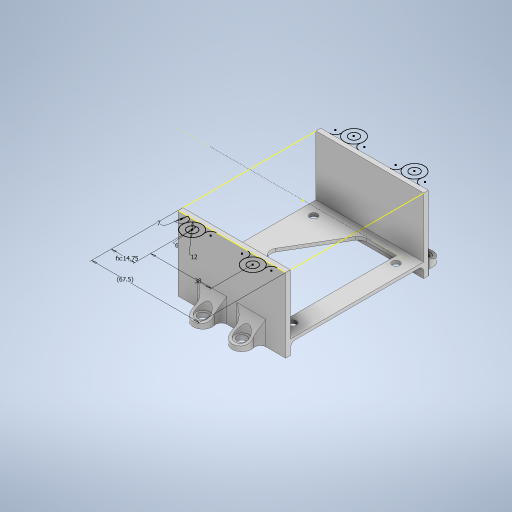
# Autodesk Inventor part: CO-1-02-fuseMount
Saved by Autodesk Inventor 2024 (Build 280153000, 153)
## iProperties
Created: 2023-03-23
Part Number: CO-1-02-fuseMount
Material: Generic
Document SubType Name: Modeling
Designer: beh5452
Density: 1 g/cm^3
Appearance: Default
Author: beh5452
Autodesk Inventor part; units mm, degrees
ref_plane "XZ Plane" through (0, 0, 0) normal (0, 1, 0) x (-1, 0, 0)
ref_plane "XY Plane" through (0, 0, 0) normal (0, 0, 1) x (1, 0, 0)
sketch "Sketch1" plane through (0, 0, 0) normal (0, 1, 0) x (-1, 0, 0)
  line L0 (33.75, 44.75) -> (-33.75, 44.75)
  line L1 (-33.75, 44.75) -> (-33.75, -44.75)
  line L2 (-33.75, -44.75) -> (33.75, -44.75)
  line L3 (33.75, -44.75) -> (33.75, 44.75)
  line L4 (21.75, -36.75) -> (-21.75, -36.75)
  line L5 (21.75, 36.75) -> (-21.75, 36.75)
  line L6 (21.75, 36.75) -> (21.75, -36.75)
  line L7 (-21.75, 36.75) -> (-21.75, -36.75)
  line L8 (33.75, -41.75) -> (-33.75, -41.75)
  line L9 (33.75, 41.75) -> (-33.75, 41.75)
  line L10 (-6.7955, 36.75) -> (21.75, 0)
  line L11 (21.75, 0) -> (0, -36.75)
  point P0 (0, 0)
  point P1 (-33.75, 0)
  dimension "d0" = 83.5
  dimension "d1" = 3
  dimension "d2" = 3
  dimension "d4" = 5
  dimension "d5" = 5
  dimension "d6" = 12
  dimension "d7" = 12
  dimension "d8" = 67.5
  dimension "d9" = 33.75
  dimension "d10" = 41.75
  constraints: 24 end point, 7 perpendicular, 5 point on line, 3 horizontal, 3 midpoint
  measures "d0" distance between parallel lines of L8 L9
  measures "d1" distance between parallel lines of L0 L9
  measures "d2" distance between parallel lines of L8 L2
  measures "d4" distance between parallel lines of L9 L5
  measures "d5" distance between parallel lines of L8 L4
  measures "d6" distance between parallel lines of L3 L6
  measures "d7" distance between parallel lines of L7 L1
  measures "d8" distance from line of point (-33.75, 0) L3
  measures "d9" distance from line of point (0, 0) L1
  measures "d10" distance from line of point (0, 0) L8
extrude "Extrusion1" add sketch "Sketch1" along normal blind 2 contours L3 L8 L1 L9 | L4 L11 L6 | L10 L5 L6
extrude "Extrusion2" add sketch "Sketch1" along normal blind 39.5 and the other way blind 7 contours L3 L9 L1 L0 | L3 L2 L1 L8
sketch "Sketch4" plane through (0, 2, 0) normal (0, 1, 0) x (1, 0, 0)
  circle A0 centre (-25.8, -32.4) radius 2.35
  circle A1 centre (-25.8, 32.4) radius 2.35
  circle A2 centre (25.8, -32.4) radius 2.35
  circle A3 centre (25.8, 32.4) radius 2.35
  line L0 (-33.75, 41.75) -> (-33.75, -41.75) projected
  line L1 (-33.75, -41.75) -> (33.75, -41.75) projected
  line L2 (33.75, -41.75) -> (33.75, 41.75) projected
  line L3 (33.75, 41.75) -> (-33.75, 41.75) projected
  point P0 (0, 0)
  dimension "d35" = 4.7
  dimension "d36" = 7.95
  dimension "d38" = 7.95
  dimension "d73" = 64.8
  dimension "d74" = 32.4
  constraints: 4 centre point, 3 equal radius, 2 horizontal alignment, 2 vertical alignment
  measures "d35" diameter of A0
  measures "d36" distance from line of L0 A0.centre
  measures "d38" distance from line of L2 A3.centre
  measures "d73" distance of A0.centre A1.centre
  measures "d74" vertical distance of point (0, 0) A0.centre
extrude "Extrusion6" cut sketch "Sketch4" against normal blind 3 contours A0 | A1 | A2 | A3
sketch "Sketch6" plane through (0, -7, 0) normal (0, -1, 0) x (1, 0, 0)
  circle A0 centre (-12.25, 50.75) radius 3
  circle A1 centre (12.25, 50.75) radius 3
  circle A2 centre (-24.5, -50.75) radius 3
  circle A3 centre (24.5, -50.75) radius 3
  circle A4 centre (-12.25, 50.75) radius 6
  circle A5 centre (-24.5, -50.75) radius 6
  circle A6 centre (24.5, -50.75) radius 6
  circle A7 centre (12.25, 50.75) radius 6
  arc A8 (-21.4152, 44.75) -> (-18.0385, 49.1711) centre (-21.4152, 48.25) ccw
  arc A9 (-6.4615, 49.1711) -> (-3.0848, 44.75) centre (-3.0848, 48.25) ccw
  arc A10 (3.0848, 44.75) -> (6.4615, 49.1711) centre (3.0848, 48.25) ccw
  arc A11 (18.0385, 49.1711) -> (21.4152, 44.75) centre (21.4152, 48.25) ccw
  arc A12 (-30.2885, -49.1711) -> (-33.6652, -44.75) centre (-33.6652, -48.25) ccw
  arc A13 (-15.3348, -44.75) -> (-18.7115, -49.1711) centre (-15.3348, -48.25) ccw
  arc A14 (18.7115, -49.1711) -> (15.3348, -44.75) centre (15.3348, -48.25) ccw
  arc A15 (33.6652, -44.75) -> (30.2885, -49.1711) centre (33.6652, -48.25) ccw
  line L0 (0, -79.45) -> (0, 79.45) projected
  circle A16 centre (0, -50.75) radius 3
  circle A17 centre (0, -50.75) radius 6
  arc A18 (9.1652, -44.75) -> (5.7885, -49.1711) centre (9.1652, -48.25) ccw
  arc A19 (-5.7885, -49.1711) -> (-9.1652, -44.75) centre (-9.1652, -48.25) ccw
  line L1 (-33.75, -44.75) -> (33.75, -44.75) projected
  line L2 (33.75, 44.75) -> (-33.75, 44.75) projected
  point P0 (0, 0)
  point P1 (-24.5, -44.75)
  point P2 (0, -44.75)
  point P3 (24.5, -44.75)
  point P4 (12.25, 44.75)
  point P5 (-12.25, 44.75)
  dimension "d46" = 6
  dimension "d47" = 6
  dimension "d48" = 6
  dimension "d49" = 6
  dimension "d51" = 12
  dimension "d54" = 3.5
  dimension "d55" = 24.5
  dimension "d56" = 49
  dimension "d57" = 12.25
  dimension "d58" = 24.5
  constraints: 30 point on circle, 25 tangent, 20 centre point, 14 equal radius, 5 coincident, 3 point on line
  measures "d46" diameter of A0
  measures "d47" diameter of A1
  measures "d48" diameter of A2
  measures "d49" diameter of A3
  measures "d51" diameter of A5
  measures "d54" radius of A12
  measures "d55" distance of A0.centre A1.centre
  measures "d56" distance of A3.centre A2.centre
  measures "d57" distance from line of L0 A1.centre
  measures "d58" distance from line of L0 A3.centre
extrude "Extrusion7" add sketch "Sketch6" against normal blind 15 contours A4 | A4 L2 A8 | A9 L2 A4 | A5 | A5 L1 A13 | A12 L1 A5 | A6 | A6 L1 A15 | A14 L1 A6 | A7 | A7 L2 A10 | A11 L2 A7 | A17 L0 A16 | L0 A16 A17 | A19 L1 A17 | L1 A18 A17
sketch "Sketch7" plane through (0, 8, 0) normal (0, 1, 0) x (1, 0, 0)
  circle A0 centre (-12.25, -50.75) radius 3 projected
  circle A1 centre (-12.25, -50.75) radius 4.25
  circle A2 centre (12.25, -50.75) radius 3 projected
  circle A3 centre (24.5, 50.75) radius 3 projected
  circle A4 centre (-24.5, 50.75) radius 3 projected
  circle A5 centre (12.25, -50.75) radius 3 projected
  circle A6 centre (12.25, -50.75) radius 4.25
  circle A7 centre (24.5, 50.75) radius 4.25
  circle A8 centre (-24.5, 50.75) radius 4.25
  circle A9 centre (0, 50.75) radius 3 projected
  circle A10 centre (0, 50.75) radius 4.25
  point P0 (0, 0)
  dimension "d61" = 8.5
  dimension "d62" = 8.5
  dimension "d63" = 8.5
  dimension "d64" = 8.5
  dimension "d72" = 8.5
  constraints: 5 centre point, 5 coincident
  measures "d61" diameter of A1
  measures "d62" diameter of A6
  measures "d63" diameter of A7
  measures "d64" diameter of A8
  measures "d72" diameter of A10
extrude "Extrusion8" cut sketch "Sketch7" against normal blind 12 contours A1 | A3 | A4 | A6 | A7 | A8 | A9 | A10
ref_plane "Work Plane1" through (30, 0, 0) normal (1, 0, 0) x (0, 1, 0)
sketch "Sketch8" plane through (30, 0, 0) normal (1, 0, 0) x (0, 1, 0)
  line L0 (-7, 56.75) -> (8, 56.75) projected
  line L1 (8, 49.1711) -> (8, 44.75) projected
  arc A0 (-4, 56.75) -> (8, 44.75) centre (8, 56.75) ccw
  line L2 (-7, 56.75) -> (-7, 44.75) projected
  line L3 (39.5, 44.75) -> (-7, 44.75) projected
  line L4 (8, 49.1711) -> (8, 56.75) projected
  arc A1 (8, -44.75) -> (-4, -56.75) centre (8, -56.75) ccw
  line L5 (8, -44.75) -> (8, -49.1711) projected
  line L6 (-7, -56.75) -> (8, -56.75) projected
  line L7 (-7, -49.1711) -> (-7, -56.75) projected
  line L8 (8, -46.5) -> (8, -55) projected
  line L9 (8, -56.75) -> (8, -49.1711) projected
  point P0 (0, 0)
  point P1 (42.5, 44.75)
  point P2 (-4, -56.75)
  dimension "d68" = 3
  dimension "d80" = 3
  constraints: 4 point on circle, 2 centre point, 1 point on line, 1 tangent
  measures "d68" distance from line of A0.start L2
  measures "d80" distance from line of L7 A1.end
extrude "Extrusion9" cut sketch "Sketch8" along normal blind 5 and the other way blind 70 contours L0 L4 L1 A0 | L5 L8 L9 L6 A1
fillet "Fillet2" radius 5 3 edges at (0, 1, -36.75) (-21.75, 1, 0) (6.7955, 1, 36.75)
fillet "Fillet7" radius 3 2 edges at (0, 0, -41.75) (0, 0, 41.75)
sketch "Sketch9" plane through (0, 39.5, 0) normal (0, 1, 0) x (1, 0, 0)
  circle A0 centre (-19, -50.75) radius 3
  circle A1 centre (-19, -50.75) radius 6
  arc A2 (-9.8348, -44.75) -> (-13.2115, -49.1711) centre (-9.8348, -48.25) ccw
  arc A3 (-24.7885, -49.1711) -> (-28.1652, -44.75) centre (-28.1652, -48.25) ccw
  line L0 (-33.75, -44.75) -> (33.75, -44.75) projected
  circle A4 centre (19, -50.75) radius 3
  circle A5 centre (19, -50.75) radius 6
  arc A6 (28.1652, -44.75) -> (24.7885, -49.1711) centre (28.1652, -48.25) ccw
  arc A7 (13.2115, -49.1711) -> (9.8348, -44.75) centre (9.8348, -48.25) ccw
  line L1 (-33.75, 41.75) -> (-33.75, -41.75) projected
  line L2 (33.75, -41.75) -> (33.75, 41.75) projected
  line L3 (-58.6769, 0) -> (43.0303, 0) construction
  line L4 (-79.0183, 0) -> (63.3717, 0) construction
  circle A8 centre (-19, 50.75) radius 3
  circle A9 centre (-19, 50.75) radius 6
  arc A10 (-13.2115, 49.1711) -> (-9.8348, 44.75) centre (-9.8348, 48.25) ccw
  arc A11 (-28.1652, 44.75) -> (-24.7885, 49.1711) centre (-28.1652, 48.25) ccw
  circle A12 centre (19, 50.75) radius 3
  circle A13 centre (19, 50.75) radius 6
  arc A14 (24.7885, 49.1711) -> (28.1652, 44.75) centre (28.1652, 48.25) ccw
  arc A15 (9.8348, 44.75) -> (13.2115, 49.1711) centre (9.8348, 48.25) ccw
  point P0 (0, 0)
  dimension "d90" = 6
  dimension "d91" = 12
  dimension "d92" = 7
  dimension "d93" = 38
  dimension "d94" = 67.5
  dimension "d95" = 14.75
  constraints: 24 point on circle, 16 centre point, 16 symmetric about line, 10 tangent, 5 equal radius, 4 coincident, 4 point on line, 2 end point, 1 collinear, 1 horizontal, 8 other
  measures "d90" diameter of A0
  measures "d91" diameter of A1
  measures "d92" diameter of A3
  measures "d93" distance of A0.centre A4.centre
  measures "d94" distance between parallel lines of L1 L2
  measures "d95" distance from line of L1 A0.centre
equation "\"d2\" = d1"
equation "\"d5\" = d4"
equation "\"d7\" = d6"
equation "\"d9\" = 0.5 * d8"
equation "\"d10\" = 0.5 * d0"
equation "\"d38\" = d36"
equation "\"d74\" = 0.5 * d73"
equation "\"d57\" = 0.5 * d55"
equation "\"d58\" = 0.5 * d56"
body "Solid1"
